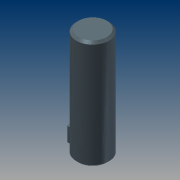
# Autodesk Inventor part: Shaft
Saved by Autodesk Inventor 2014 (Build 180170000, 170)
## iProperties
Created: 2021-03-18
Part Number: Shaft
Material: Lead
Document SubType Name: Modeling
Designer: Think Station
Density: 11.37 g/cm^3
Appearance: Lead
Author: Think Station
Autodesk Inventor part; units mm, degrees
ref_plane "XZ Plane" through (0, 0, 0) normal (0, 1, 0) x (-1, 0, 0)
ref_plane "XY Plane" through (0, 0, 0) normal (0, 0, 1) x (1, 0, 0)
sketch "Sketch1" plane through (0, 0, 0) normal (0, 0, 1) x (1, 0, 0)
  circle A0 centre (0, 0) radius 15
  dimension "d0" = 30
  constraints: 1 centre point, 1 coincident
  measures "d0" diameter of A0
extrude "Extrusion1" add sketch "Sketch1" along normal blind 100
chamfer "Chamfer1" distance 2 angle 45 1 edges at (-15, 0, 100)
chamfer "Chamfer2" distance 2 angle 45 1 edges at (-15, 0, 0)
ref_plane "Work Plane1" through (-10, 0, 0) normal (1, 0, 0) x (0, 1, 0)
sketch "Sketch2" plane through (-10, 0, 0) normal (1, 0, 0) x (0, 1, 0)
  line L0 (-15, 2) -> (15, 2) projected
  line L1 (4, 2) -> (-4, 2)
  line L2 (-4, 2) -> (-4, 15)
  line L3 (-4, 15) -> (4, 15)
  line L4 (4, 15) -> (4, 2)
  line L5 (4, 2) -> (-4, 15) construction
  line L6 (-4, 2) -> (4, 15) construction
  line L7 (0, -20) -> (0, 120) projected
  line L8 (15, 98) -> (-15, 98) projected
  line L9 (-15, 2) -> (15, 2) projected
  line L10 (-15, 2) -> (-15, 98) projected
  line L11 (15, 2) -> (15, 98) projected
  point P0 (0, 0)
  point P1 (0, 8.5)
  dimension "d10" = 8
  dimension "d11" = 13
  dimension "d12" = 15
  constraints: 12 end point, 2 midpoint, 2 parallel, 1 collinear, 1 horizontal, 1 perpendicular
  measures "d10" distance of L2.end L3.end
  measures "d11" distance of L1.end L2.end
  measures "d12" distance from line of L11 point (0, 8.5)
extrude "Extrusion2" add sketch "Sketch2" against normal blind 10 contours L2 L3 L7 L0 | L7 L3 L4 L0
fillet "Fillet1" radius 1 2 edges at (-20, 4, 8.5) (-20, -4, 8.5)
body "Solid1"
